Autodesk Inventor part; units mm, degrees
(part 2 of 5)
  line L413 (269.721, 22.163) -> (269.721, 35.9625) projected
  line L414 (269.721, 35.9625) -> (283.52, 35.9625) projected
  line L415 (269.721, 35.9625) -> (283.52, 35.9625) projected
  line L416 (279.888, 47.7132) -> (279.888, 41.4433) projected
  line L417 (279.888, 47.7132) -> (279.888, 41.4433) projected
  line L418 (280.713, 47.7132) -> (279.888, 47.7132) projected
  line L419 (280.713, 47.7132) -> (279.888, 47.7132) projected
  line L420 (302.57, 55.0125) -> (302.57, 41.2129) projected
  line L421 (302.57, 55.0125) -> (302.57, 41.2129) projected
  line L422 (280.713, 50.3135) -> (280.713, 47.7132) projected
  line L423 (280.713, 50.3135) -> (280.713, 47.7132) projected
  line L424 (279.888, 50.3135) -> (280.713, 50.3135) projected
  line L425 (279.888, 50.3135) -> (280.713, 50.3135) projected
  line L426 (279.888, 53.5421) -> (279.888, 50.3135) projected
  line L427 (279.888, 53.5421) -> (279.888, 50.3135) projected
  line L428 (288.771, 41.2129) -> (288.771, 55.0125) projected
  line L429 (288.771, 41.2129) -> (288.771, 55.0125) projected
  line L430 (288.771, 55.0125) -> (302.57, 55.0125) projected
  line L431 (288.771, 55.0125) -> (302.57, 55.0125) projected
  line L432 (302.57, 41.2129) -> (288.771, 41.2129) projected
  line L433 (302.57, 41.2129) -> (288.771, 41.2129) projected
  line L434 (305.398, 1.5696) -> (305.441, 1.7198) projected
  line L435 (305.278, 1.2788) -> (305.343, 1.4221) projected
  line L436 (305.114, 1.0115) -> (305.201, 1.1424) projected
  line L437 (305.343, 1.4221) -> (305.398, 1.5696) projected
  line L438 (305.016, 0.8875) -> (305.114, 1.0115) projected
  line L439 (305.441, 1.7198) -> (305.471, 1.8741) projected
  line L440 (305.471, 1.8741) -> (305.489, 2.0298) projected
  line L441 (305.489, 2.0298) -> (305.496, 2.1869) projected
  line L442 (305.016, 0.8875) -> (305.114, 1.0115) projected
  line L443 (305.016, 0.8875) -> (305.114, 1.0115) projected
  line L444 (305.016, 0.8875) -> (305.114, 1.0115) projected
  line L445 (305.114, 1.0115) -> (305.201, 1.1424) projected
  line L446 (305.114, 1.0115) -> (305.201, 1.1424) projected
  line L447 (305.114, 1.0115) -> (305.201, 1.1424) projected
  line L448 (305.201, 1.1424) -> (305.278, 1.2788) projected
  line L449 (305.201, 1.1424) -> (305.278, 1.2788) projected
  line L450 (305.201, 1.1424) -> (305.278, 1.2788) projected
  line L451 (305.278, 1.2788) -> (305.343, 1.4221) projected
  line L452 (305.278, 1.2788) -> (305.343, 1.4221) projected
  line L453 (305.278, 1.2788) -> (305.343, 1.4221) projected
  line L454 (305.343, 1.4221) -> (305.398, 1.5696) projected
  line L455 (305.343, 1.4221) -> (305.398, 1.5696) projected
  line L456 (305.343, 1.4221) -> (305.398, 1.5696) projected
  line L457 (305.398, 1.5696) -> (305.441, 1.7198) projected
  line L458 (305.398, 1.5696) -> (305.441, 1.7198) projected
  line L459 (305.398, 1.5696) -> (305.441, 1.7198) projected
  line L460 (305.441, 1.7198) -> (305.471, 1.8741) projected
  line L461 (305.441, 1.7198) -> (305.471, 1.8741) projected
  line L462 (305.441, 1.7198) -> (305.471, 1.8741) projected
  line L463 (305.471, 1.8741) -> (305.489, 2.0298) projected
  line L464 (305.471, 1.8741) -> (305.489, 2.0299) projected
  line L465 (305.471, 1.8741) -> (305.489, 2.0298) projected
  line L466 (305.489, 2.0298) -> (305.496, 2.1869) projected
  line L467 (305.489, 2.0299) -> (305.496, 2.1869) projected
  line L468 (305.489, 2.0298) -> (305.496, 2.187) projected
  line L469 (304.115, 0.2853) -> (304.261, 0.339) projected
  line L470 (250.671, 16.9127) -> (264.47, 16.9127) projected
  line L471 (250.671, 16.9127) -> (264.47, 16.9127) projected
  line L472 (264.47, 16.9127) -> (264.47, 3.113) projected
  line L473 (264.47, 16.9127) -> (264.47, 3.113) projected
  line L474 (264.47, 3.113) -> (250.671, 3.113) projected
  line L475 (264.47, 3.113) -> (250.671, 3.113) projected
  line L476 (269.721, 16.9127) -> (283.52, 16.9127) projected
  line L477 (269.721, 16.9127) -> (283.52, 16.9127) projected
  line L478 (283.52, 16.9127) -> (283.52, 3.113) projected
  line L479 (283.52, 3.113) -> (269.721, 3.113) projected
  line L480 (283.52, 3.113) -> (269.721, 3.113) projected
  line L481 (269.721, 3.113) -> (269.721, 16.9127) projected
  line L482 (269.721, 3.113) -> (269.721, 16.9127) projected
  line L483 (283.52, 16.9127) -> (283.52, 3.113) projected
  line L484 (243.527, 35.9625) -> (257.327, 35.9625) projected
  line L485 (243.527, 35.9625) -> (257.327, 35.9625) projected
  line L486 (257.327, 35.9625) -> (257.327, 22.163) projected
  line L487 (257.327, 35.9625) -> (257.327, 22.163) projected
  line L488 (257.327, 22.163) -> (243.527, 22.163) projected
  line L489 (233.514, 16.9127) -> (233.514, 3.113) projected
  line L490 (233.514, 16.9127) -> (233.514, 3.113) projected
  line L491 (257.327, 22.163) -> (243.527, 22.163) projected
  line L492 (250.671, 3.113) -> (250.671, 16.9127) projected
  line L493 (250.671, 3.113) -> (250.671, 16.9127) projected
  line L494 (233.514, 3.113) -> (219.713, 3.113) projected
  line L495 (233.514, 3.113) -> (219.713, 3.113) projected
  line L496 (219.713, 3.113) -> (219.713, 16.9127) projected
  line L497 (219.713, 3.113) -> (219.713, 16.9127) projected
  line L498 (243.527, 22.163) -> (243.527, 35.9625) projected
  line L499 (243.527, 22.163) -> (243.527, 35.9625) projected
  line L500 (219.713, 16.9127) -> (233.514, 16.9127) projected
  line L501 (219.713, 16.9127) -> (233.514, 16.9127) projected
  line L502 (231.133, 35.9625) -> (231.133, 22.163) projected
  line L503 (231.133, 35.9625) -> (231.133, 22.163) projected
  line L504 (231.133, 22.163) -> (217.333, 22.163) projected
  line L505 (231.133, 22.163) -> (217.333, 22.163) projected
  line L506 (217.333, 35.9625) -> (231.133, 35.9625) projected
  line L507 (217.333, 35.9625) -> (231.133, 35.9625) projected
  line L508 (217.333, 22.163) -> (217.333, 35.9625) projected
  line L509 (217.333, 22.163) -> (217.333, 35.9625) projected
  line L510 (241.146, 60.2629) -> (241.146, 74.0625) projected
  line L511 (1.6288, 119.796) -> (1.4759, 119.753) projected
  line L512 (1.4759, 119.753) -> (1.3298, 119.698) projected
  line L513 (1.3298, 119.698) -> (1.1879, 119.633) projected
  line L514 (1.3298, 119.698) -> (1.1879, 119.633) projected
  line L515 (1.1879, 119.633) -> (1.0501, 119.556) projected
  line L516 (1.1879, 119.633) -> (1.0501, 119.556) projected
  line L517 (1.0501, 119.556) -> (0.9192, 119.469) projected
  line L518 (1.0501, 119.556) -> (0.9192, 119.469) projected
  line L519 (1.4759, 119.753) -> (1.3298, 119.698) projected
  line L520 (1.6288, 119.796) -> (1.4759, 119.753) projected
  line L521 (0.9192, 119.469) -> (0.7965, 119.371) projected
  line L522 (0.7965, 119.371) -> (0.6808, 119.265) projected
  line L523 (0.7965, 119.371) -> (0.6808, 119.265) projected
  line L524 (0.6808, 119.265) -> (0.5746, 119.149) projected
  line L525 (0.6808, 119.265) -> (0.5746, 119.149) projected
  line L526 (0.5746, 119.149) -> (0.4768, 119.025) projected
  line L527 (0.5746, 119.149) -> (0.4768, 119.025) projected
  line L528 (0.4768, 119.025) -> (0.39, 118.894) projected
  line L529 (0.4768, 119.025) -> (0.39, 118.894) projected
  line L530 (303.496, 119.849) -> (2.096, 119.849) projected
  line L531 (303.496, 119.849) -> (2.096, 119.849) projected
  line L532 (2.096, 119.849) -> (1.9389, 119.844) projected
  line L533 (2.096, 119.849) -> (1.9389, 119.844) projected
  line L534 (1.9389, 119.844) -> (1.7818, 119.826) projected
  line L535 (1.9389, 119.844) -> (1.7818, 119.826) projected
  line L536 (1.7818, 119.826) -> (1.6288, 119.796) projected
  line L537 (1.7818, 119.826) -> (1.6288, 119.796) projected
  line L538 (303.496, 119.849) -> (2.096, 119.849) projected
  line L539 (303.496, 119.849) -> (2.096, 119.849) projected
  line L540 (303.496, 119.849) -> (2.096, 119.849) projected
  line L541 (2.096, 119.849) -> (1.9389, 119.844) projected
  line L542 (1.9389, 119.844) -> (1.7818, 119.826) projected
  line L543 (1.7818, 119.826) -> (1.6288, 119.796) projected
  line L544 (1.6288, 119.796) -> (1.4759, 119.753) projected
  line L545 (1.4759, 119.753) -> (1.3298, 119.698) projected
  line L546 (1.3298, 119.698) -> (1.1879, 119.633) projected
  line L547 (1.1879, 119.633) -> (1.0501, 119.556) projected
  line L548 (1.0501, 119.556) -> (0.9192, 119.469) projected
  line L549 (0.9192, 119.469) -> (0.7965, 119.371) projected
  line L550 (0.7965, 119.371) -> (0.6808, 119.265) projected
  line L551 (0.6808, 119.265) -> (0.5746, 119.149) projected
  line L552 (0.5746, 119.149) -> (0.4768, 119.025) projected
  line L553 (0.4768, 119.025) -> (0.39, 118.894) projected
  line L554 (0.39, 118.894) -> (0.3128, 118.758) projected
  line L555 (0.3128, 118.758) -> (0.248, 118.616) projected
  line L556 (0.248, 118.616) -> (0.1929, 118.468) projected
  line L557 (0.1929, 118.468) -> (0.1502, 118.317) projected
  line L558 (0.1502, 118.317) -> (0.1199, 118.163) projected
  line L559 (0.1199, 118.163) -> (0.102, 118.007) projected
  line L560 (0.102, 118.007) -> (0.0951, 117.85) projected
  line L561 (0.0951, 117.85) -> (0.0951, 2.187) projected
  line L562 (0.0951, 2.187) -> (0.102, 2.0298) projected
  line L563 (0.102, 2.0298) -> (0.1199, 1.8741) projected
  line L564 (0.1199, 1.8741) -> (0.1502, 1.7198) projected
  line L565 (0.1502, 1.7198) -> (0.1929, 1.5696) projected
  line L566 (0.1929, 1.5696) -> (0.248, 1.4221) projected
  line L567 (0.248, 1.4221) -> (0.3128, 1.2788) projected
  line L568 (0.3128, 1.2788) -> (0.39, 1.1424) projected
  line L569 (0.39, 1.1424) -> (0.4768, 1.0115) projected
  line L570 (0.4768, 1.0115) -> (0.5746, 0.8875) projected
  line L571 (0.5746, 0.8875) -> (0.6808, 0.7731) projected
  line L572 (0.6808, 0.7731) -> (0.7965, 0.6656) projected
  line L573 (0.7965, 0.6656) -> (0.9192, 0.5691) projected
  line L574 (0.9192, 0.5691) -> (1.0501, 0.4823) projected
  line L575 (1.0501, 0.4823) -> (1.1879, 0.4051) projected
  line L576 (1.1879, 0.4051) -> (1.3298, 0.339) projected
  line L577 (1.3298, 0.339) -> (1.4759, 0.2853) projected
  line L578 (1.4759, 0.2853) -> (1.6288, 0.2425) projected
  line L579 (1.6288, 0.2425) -> (1.7818, 0.2122) projected
  line L580 (1.7818, 0.2122) -> (1.9389, 0.1929) projected
  line L581 (1.9389, 0.1929) -> (2.096, 0.1874) projected
  line L582 (2.096, 0.1874) -> (303.496, 0.1874) projected
  line L583 (303.496, 0.1874) -> (303.652, 0.1929) projected
  line L584 (303.652, 0.1929) -> (303.808, 0.2122) projected
  line L585 (303.808, 0.2122) -> (303.962, 0.2425) projected
  line L586 (303.962, 0.2425) -> (304.115, 0.2853) projected
  line L587 (304.115, 0.2853) -> (304.261, 0.339) projected
  line L588 (304.261, 0.339) -> (304.403, 0.4051) projected
  line L589 (304.403, 0.4051) -> (304.541, 0.4823) projected
  line L590 (304.541, 0.4823) -> (304.672, 0.5691) projected
  line L591 (304.672, 0.5691) -> (304.794, 0.6656) projected
  line L592 (304.794, 0.6656) -> (304.91, 0.7731) projected
  line L593 (304.91, 0.7731) -> (305.016, 0.8875) projected
  line L594 (305.016, 0.8875) -> (305.114, 1.0115) projected
  line L595 (305.114, 1.0115) -> (305.201, 1.1424) projected
  line L596 (305.201, 1.1424) -> (305.278, 1.2788) projected
  line L597 (305.278, 1.2788) -> (305.343, 1.4221) projected
  line L598 (305.343, 1.4221) -> (305.398, 1.5696) projected
  line L599 (305.398, 1.5696) -> (305.441, 1.7198) projected
  line L600 (305.441, 1.7198) -> (305.471, 1.8741) projected
  line L601 (305.471, 1.8741) -> (305.489, 2.0298) projected
  line L602 (305.489, 2.0298) -> (305.496, 2.187) projected
  line L603 (305.496, 2.187) -> (305.496, 117.85) projected
  line L604 (305.496, 117.85) -> (305.489, 118.007) projected
  line L605 (305.489, 118.007) -> (305.471, 118.163) projected
  line L606 (305.471, 118.163) -> (305.441, 118.317) projected
  line L607 (305.441, 118.317) -> (305.398, 118.468) projected
  line L608 (305.398, 118.468) -> (305.343, 118.616) projected
  line L609 (305.343, 118.616) -> (305.278, 118.758) projected
  line L610 (305.278, 118.758) -> (305.201, 118.894) projected
  line L611 (305.201, 118.894) -> (305.114, 119.025) projected
  line L612 (305.114, 119.025) -> (305.016, 119.149) projected
  line L613 (305.016, 119.149) -> (304.91, 119.265) projected
  line L614 (304.91, 119.265) -> (304.794, 119.371) projected
  line L615 (304.794, 119.371) -> (304.672, 119.469) projected
  line L616 (304.672, 119.469) -> (304.541, 119.556) projected
  line L617 (304.541, 119.556) -> (304.403, 119.633) projected
  line L618 (304.403, 119.633) -> (304.261, 119.698) projected
  line L619 (304.261, 119.698) -> (304.115, 119.753) projected
  line L620 (304.115, 119.753) -> (303.962, 119.796) projected
  line L621 (303.962, 119.796) -> (303.808, 119.826) projected
  line L622 (303.808, 119.826) -> (303.652, 119.844) projected
  line L623 (303.652, 119.844) -> (303.496, 119.849) projected
  line L624 (288.771, 79.3129) -> (288.771, 93.1125) projected
  line L625 (288.771, 93.1125) -> (302.57, 93.1125) projected
  line L626 (302.57, 93.1125) -> (302.57, 79.3129) projected
  line L627 (302.57, 79.3129) -> (288.771, 79.3129) projected
  line L628 (243.527, 35.9625) -> (257.327, 35.9625) projected
  line L629 (257.327, 35.9625) -> (257.327, 22.163) projected
  line L630 (257.327, 22.163) -> (243.527, 22.163) projected
  line L631 (243.527, 22.163) -> (243.527, 35.9625) projected
  line L632 (302.57, 60.2629) -> (288.771, 60.2629) projected
  line L633 (288.771, 60.2629) -> (288.771, 74.0625) projected
  line L634 (288.771, 74.0625) -> (302.57, 74.0625) projected
  line L635 (302.57, 74.0625) -> (302.57, 60.2629) projected
  line L636 (250.671, 16.9127) -> (264.47, 16.9127) projected
  line L637 (264.47, 16.9127) -> (264.47, 3.113) projected
  line L638 (264.47, 3.113) -> (250.671, 3.113) projected
  line L639 (250.671, 3.113) -> (250.671, 16.9127) projected
  line L640 (219.713, 16.9127) -> (233.514, 16.9127) projected
  line L641 (233.514, 16.9127) -> (233.514, 3.113) projected
  line L642 (233.514, 3.113) -> (219.713, 3.113) projected
  line L643 (219.713, 3.113) -> (219.713, 16.9127) projected
  line L644 (302.57, 41.2129) -> (288.771, 41.2129) projected
  line L645 (288.771, 41.2129) -> (288.771, 55.0125) projected
  line L646 (288.771, 55.0125) -> (302.57, 55.0125) projected
  line L647 (302.57, 55.0125) -> (302.57, 41.2129) projected
  line L648 (288.771, 16.9127) -> (302.57, 16.9127) projected
  line L649 (302.57, 16.9127) -> (302.57, 3.113) projected
  line L650 (302.57, 3.113) -> (288.771, 3.113) projected
  line L651 (288.771, 3.113) -> (288.771, 16.9127) projected
  line L652 (269.721, 16.9127) -> (283.52, 16.9127) projected
  line L653 (283.52, 16.9127) -> (283.52, 3.113) projected
  line L654 (283.52, 3.113) -> (269.721, 3.113) projected
  line L655 (269.721, 3.113) -> (269.721, 16.9127) projected
  line L656 (283.52, 22.163) -> (269.721, 22.163) projected
  line L657 (269.721, 22.163) -> (269.721, 35.9625) projected
  line L658 (269.721, 35.9625) -> (283.52, 35.9625) projected
  line L659 (283.52, 35.9625) -> (283.52, 22.163) projected
  line L660 (288.771, 35.9625) -> (302.57, 35.9625) projected
  line L661 (302.57, 35.9625) -> (302.57, 22.163) projected
  line L662 (302.57, 22.163) -> (288.771, 22.163) projected
  line L663 (288.771, 22.163) -> (288.771, 35.9625) projected
  line L664 (59.6829, 35.9625) -> (59.6829, 22.163) projected
  line L665 (59.6829, 22.163) -> (45.8833, 22.163) projected
  line L666 (45.8833, 22.163) -> (45.8833, 35.9625) projected
  line L667 (45.8833, 35.9625) -> (59.6829, 35.9625) projected
  line L668 (5.4019, 16.9127) -> (19.2016, 16.9127) projected
  line L669 (19.2016, 16.9127) -> (19.2016, 3.113) projected
  line L670 (19.2016, 3.113) -> (5.4019, 3.113) projected
  line L671 (5.4019, 3.113) -> (5.4019, 16.9127) projected
  line L672 (29.213, 16.9127) -> (43.0142, 16.9127) projected
  line L673 (43.0142, 16.9127) -> (43.0142, 3.113) projected
  line L674 (43.0142, 3.113) -> (29.213, 3.113) projected
  line L675 (29.213, 3.113) -> (29.213, 16.9127) projected
  line L676 (145.408, 55.0125) -> (145.408, 41.2129) projected
  line L677 (145.408, 41.2129) -> (131.608, 41.2129) projected
  line L678 (131.608, 41.2129) -> (131.608, 55.0125) projected
  line L679 (131.608, 55.0125) -> (145.408, 55.0125) projected
  line L680 (164.458, 41.2129) -> (150.658, 41.2129) projected
  line L681 (150.658, 41.2129) -> (150.658, 55.0125) projected
  line L682 (150.658, 55.0125) -> (164.458, 55.0125) projected
  line L683 (164.458, 55.0125) -> (164.458, 41.2129) projected
  line L684 (273.995, 103.125) -> (260.196, 103.125) projected
  line L685 (260.196, 103.125) -> (260.196, 116.926) projected
  line L686 (260.196, 116.926) -> (273.995, 116.926) projected
  line L687 (273.995, 116.926) -> (273.995, 103.125) projected
  line L688 (241.146, 74.0625) -> (254.945, 74.0625) projected
  line L689 (254.945, 74.0625) -> (254.945, 60.2629) projected
  line L690 (254.945, 60.2629) -> (241.146, 60.2629) projected
  line L691 (241.146, 60.2629) -> (241.146, 74.0625) projected
  line L692 (254.945, 103.125) -> (241.146, 103.125) projected
  line L693 (241.146, 103.125) -> (241.146, 116.926) projected
  line L694 (241.146, 116.926) -> (254.945, 116.926) projected
  line L695 (254.945, 116.926) -> (254.945, 103.125) projected
  line L696 (235.895, 103.125) -> (222.096, 103.125) projected
  line L697 (222.096, 103.125) -> (222.096, 116.926) projected
  line L698 (222.096, 116.926) -> (235.895, 116.926) projected
  line L699 (235.895, 116.926) -> (235.895, 103.125) projected
  line L700 (245.42, 79.3129) -> (231.621, 79.3129) projected
  line L701 (231.621, 79.3129) -> (231.621, 93.1125) projected
  line L702 (231.621, 93.1125) -> (245.42, 93.1125) projected
  line L703 (245.42, 93.1125) -> (245.42, 79.3129) projected
  line L704 (226.37, 79.3129) -> (212.571, 79.3129) projected
  line L705 (212.571, 79.3129) -> (212.571, 93.1125) projected
  line L706 (212.571, 93.1125) -> (226.37, 93.1125) projected
  line L707 (226.37, 93.1125) -> (226.37, 79.3129) projected
  line L708 (217.333, 35.9625) -> (231.133, 35.9625) projected
  line L709 (231.133, 35.9625) -> (231.133, 22.163) projected
  line L710 (231.133, 22.163) -> (217.333, 22.163) projected
  line L711 (217.333, 22.163) -> (217.333, 35.9625) projected
  line L712 (198.283, 35.9625) -> (212.083, 35.9625) projected
  line L713 (212.083, 35.9625) -> (212.083, 22.163) projected
  line L714 (212.083, 22.163) -> (198.283, 22.163) projected
  line L715 (198.283, 22.163) -> (198.283, 35.9625) projected
  line L716 (235.895, 60.2629) -> (222.096, 60.2629) projected
  line L717 (222.096, 60.2629) -> (222.096, 74.0625) projected
  line L718 (222.096, 74.0625) -> (235.895, 74.0625) projected
  line L719 (235.895, 74.0625) -> (235.895, 60.2629) projected
  line L720 (193.033, 103.125) -> (179.233, 103.125) projected
  line L721 (179.233, 103.125) -> (179.233, 116.926) projected
  line L722 (179.233, 116.926) -> (193.033, 116.926) projected
  line L723 (193.033, 116.926) -> (193.033, 103.125) projected
  line L724 (216.845, 103.125) -> (203.046, 103.125) projected
  line L725 (203.046, 103.125) -> (203.046, 116.926) projected
  line L726 (203.046, 116.926) -> (216.845, 116.926) projected
  line L727 (216.845, 116.926) -> (216.845, 103.125) projected
  line L728 (216.845, 74.0625) -> (216.845, 60.2629) projected
  line L729 (216.845, 60.2629) -> (203.046, 60.2629) projected
  line L730 (203.046, 60.2629) -> (203.046, 74.0625) projected
  line L731 (203.046, 74.0625) -> (216.845, 74.0625) projected
  line L732 (207.32, 79.3129) -> (193.521, 79.3129) projected
  line L733 (193.521, 79.3129) -> (193.521, 93.1125) projected
  line L734 (193.521, 93.1125) -> (207.32, 93.1125) projected
  line L735 (207.32, 93.1125) -> (207.32, 79.3129) projected
  line L736 (188.27, 79.3129) -> (174.471, 79.3129) projected
  line L737 (174.471, 79.3129) -> (174.471, 93.1125) projected
  line L738 (174.471, 93.1125) -> (188.27, 93.1125) projected
  line L739 (188.27, 93.1125) -> (188.27, 79.3129) projected
  line L740 (183.508, 55.0125) -> (183.508, 41.2129) projected
  line L741 (183.508, 41.2129) -> (169.708, 41.2129) projected
  line L742 (169.708, 41.2129) -> (169.708, 55.0125) projected
  line L743 (169.708, 55.0125) -> (183.508, 55.0125) projected
  line L744 (197.795, 60.2629) -> (183.996, 60.2629) projected
  line L745 (183.996, 60.2629) -> (183.996, 74.0625) projected
  line L746 (183.996, 74.0625) -> (197.795, 74.0625) projected
  line L747 (197.795, 74.0625) -> (197.795, 60.2629) projected
  line L748 (178.745, 74.0625) -> (178.745, 60.2629) projected
  line L749 (178.745, 60.2629) -> (164.946, 60.2629) projected
  line L750 (164.946, 60.2629) -> (164.946, 74.0625) projected
  line L751 (164.946, 74.0625) -> (178.745, 74.0625) projected
  line L752 (154.933, 103.125) -> (141.133, 103.125) projected
  line L753 (141.133, 103.125) -> (141.133, 116.926) projected
  line L754 (141.133, 116.926) -> (154.933, 116.926) projected
  line L755 (154.933, 116.926) -> (154.933, 103.125) projected
  line L756 (173.983, 103.125) -> (160.183, 103.125) projected
  line L757 (160.183, 103.125) -> (160.183, 116.926) projected
  line L758 (160.183, 116.926) -> (173.983, 116.926) projected
  line L759 (173.983, 116.926) -> (173.983, 103.125) projected
  line L760 (169.22, 79.3129) -> (155.421, 79.3129) projected
  line L761 (155.421, 79.3129) -> (155.421, 93.1125) projected
  line L762 (155.421, 93.1125) -> (169.22, 93.1125) projected
  line L763 (169.22, 93.1125) -> (169.22, 79.3129) projected
  line L764 (150.17, 79.3129) -> (136.371, 79.3129) projected
  line L765 (136.371, 79.3129) -> (136.371, 93.1125) projected
  line L766 (136.371, 93.1125) -> (150.17, 93.1125) projected
  line L767 (150.17, 93.1125) -> (150.17, 79.3129) projected
  line L768 (260.196, 79.3129) -> (260.196, 84.0133) projected
  line L769 (260.196, 84.0133) -> (258.47, 84.0133) projected
  line L770 (258.47, 84.0133) -> (258.47, 79.5433) projected
  line L771 (258.47, 79.5433) -> (256.745, 79.5433) projected
  line L772 (256.745, 79.5433) -> (256.745, 78.3428) projected
  line L773 (256.745, 78.3428) -> (253.646, 78.3428) projected
  line L774 (253.646, 78.3428) -> (253.646, 79.5433) projected
  line L775 (253.646, 79.5433) -> (251.92, 79.5433) projected
  line L776 (251.92, 79.5433) -> (251.92, 85.8132) projected
  line L777 (251.92, 85.8132) -> (251.095, 85.8132) projected
  line L778 (251.095, 85.8132) -> (251.095, 88.4135) projected
  line L779 (251.095, 88.4135) -> (251.92, 88.4135) projected
  line L780 (251.92, 88.4135) -> (251.92, 91.6421) projected
  line L781 (251.92, 91.6421) -> (258.47, 91.6421) projected
  line L782 (258.47, 91.6421) -> (258.47, 88.4135) projected
  line L783 (258.47, 88.4135) -> (260.196, 88.4135) projected
  line L784 (260.196, 88.4135) -> (260.196, 93.1125) projected
  line L785 (260.196, 93.1125) -> (273.995, 93.1125) projected
  line L786 (273.995, 93.1125) -> (273.995, 88.4135) projected
  line L787 (273.995, 88.4135) -> (275.721, 88.4135) projected
  line L788 (275.721, 88.4135) -> (275.721, 91.6421) projected
  line L789 (275.721, 91.6421) -> (282.271, 91.6421) projected
  line L790 (282.271, 91.6421) -> (282.271, 88.4135) projected
  line L791 (282.271, 88.4135) -> (283.096, 88.4135) projected
  line L792 (283.096, 88.4135) -> (283.096, 85.8132) projected
  line L793 (283.096, 85.8132) -> (282.271, 85.8132) projected
  line L794 (282.271, 85.8132) -> (282.271, 79.5433) projected
  line L795 (282.271, 79.5433) -> (280.545, 79.5433) projected
  line L796 (280.545, 79.5433) -> (280.545, 78.3428) projected
  line L797 (280.545, 78.3428) -> (277.446, 78.3428) projected
  line L798 (277.446, 78.3428) -> (277.446, 79.5433) projected
  line L799 (277.446, 79.5433) -> (275.721, 79.5433) projected
  line L800 (275.721, 79.5433) -> (275.721, 84.0133) projected
  line L801 (275.721, 84.0133) -> (273.995, 84.0133) projected
  line L802 (273.995, 84.0133) -> (273.995, 79.3129) projected
  line L803 (273.995, 79.3129) -> (260.196, 79.3129) projected
  line L804 (278.758, 60.2629) -> (264.958, 60.2629) projected
  line L805 (264.958, 60.2629) -> (264.958, 74.0625) projected
  line L806 (264.958, 74.0625) -> (278.758, 74.0625) projected
  line L807 (278.758, 74.0625) -> (278.758, 60.2629) projected
  line L808 (257.813, 55.0125) -> (271.614, 55.0125) projected
  line L809 (271.614, 55.0125) -> (271.614, 50.3135) projected
  line L810 (271.614, 50.3135) -> (273.338, 50.3135) projected
  line L811 (273.338, 50.3135) -> (273.338, 53.5421) projected
  line L812 (273.338, 53.5421) -> (279.888, 53.5421) projected
  line L813 (279.888, 53.5421) -> (279.888, 50.3135) projected
  line L814 (279.888, 50.3135) -> (280.713, 50.3135) projected
  line L815 (280.713, 50.3135) -> (280.713, 47.7132) projected
  line L816 (280.713, 47.7132) -> (279.888, 47.7132) projected
  line L817 (279.888, 47.7132) -> (279.888, 41.4433) projected
  line L818 (279.888, 41.4433) -> (278.164, 41.4433) projected
  line L819 (278.164, 41.4433) -> (278.164, 40.2428) projected
  line L820 (278.164, 40.2428) -> (275.063, 40.2428) projected
  line L821 (275.063, 40.2428) -> (275.063, 41.4433) projected
  line L822 (275.063, 41.4433) -> (273.338, 41.4433) projected
  line L823 (273.338, 41.4433) -> (273.338, 45.9133) projected
  line L824 (273.338, 45.9133) -> (271.614, 45.9133) projected
  line L825 (271.614, 45.9133) -> (271.614, 41.2129) projected
  line L826 (271.614, 41.2129) -> (257.813, 41.2129) projected
  line L827 (257.813, 41.2129) -> (257.813, 45.9133) projected
  line L828 (257.813, 45.9133) -> (256.089, 45.9133) projected
  line L829 (256.089, 45.9133) -> (256.089, 41.4433) projected
  line L830 (256.089, 41.4433) -> (254.362, 41.4433) projected
  line L831 (254.362, 41.4433) -> (254.362, 40.2428) projected
  line L832 (254.362, 40.2428) -> (251.263, 40.2428) projected
  line L833 (251.263, 40.2428) -> (251.263, 41.4433) projected
  line L834 (251.263, 41.4433) -> (249.538, 41.4433) projected
  line L835 (249.538, 41.4433) -> (249.538, 47.7132) projected
  line L836 (249.538, 47.7132) -> (248.714, 47.7132) projected
  line L837 (248.714, 47.7132) -> (248.714, 50.3135) projected
  line L838 (248.714, 50.3135) -> (249.538, 50.3135) projected
  line L839 (249.538, 50.3135) -> (249.538, 53.5421) projected
  line L840 (249.538, 53.5421) -> (256.089, 53.5421) projected
  line L841 (256.089, 53.5421) -> (256.089, 50.3135) projected
  line L842 (256.089, 50.3135) -> (257.813, 50.3135) projected
  line L843 (257.813, 50.3135) -> (257.813, 55.0125) projected
  line L844 (226.858, 41.2129) -> (226.858, 55.0125) projected
  line L845 (226.858, 55.0125) -> (240.658, 55.0125) projected
  line L846 (240.658, 55.0125) -> (240.658, 41.2129) projected
  line L847 (240.658, 41.2129) -> (226.858, 41.2129) projected
  line L848 (221.608, 55.0125) -> (221.608, 41.2129) projected
  line L849 (221.608, 41.2129) -> (207.808, 41.2129) projected
  line L850 (207.808, 41.2129) -> (207.808, 55.0125) projected
  line L851 (207.808, 55.0125) -> (221.608, 55.0125) projected
  line L852 (202.558, 41.2129) -> (188.758, 41.2129) projected
  line L853 (188.758, 41.2129) -> (188.758, 55.0125) projected
  line L854 (188.758, 55.0125) -> (202.558, 55.0125) projected
  line L855 (202.558, 55.0125) -> (202.558, 41.2129) projected
  line L856 (122.083, 35.9625) -> (135.883, 35.9625) projected
  line L857 (135.883, 35.9625) -> (135.883, 22.163) projected
  line L858 (135.883, 22.163) -> (122.083, 22.163) projected
  line L859 (122.083, 22.163) -> (122.083, 35.9625) projected
  line L860 (195.902, 16.9127) -> (209.702, 16.9127) projected
  line L861 (209.702, 16.9127) -> (209.702, 3.113) projected
  line L862 (209.702, 3.113) -> (195.902, 3.113) projected
  line L863 (195.902, 3.113) -> (195.902, 16.9127) projected
  line L864 (193.033, 22.163) -> (179.233, 22.163) projected
  line L865 (179.233, 22.163) -> (179.233, 35.9625) projected
  line L866 (179.233, 35.9625) -> (193.033, 35.9625) projected
  line L867 (193.033, 35.9625) -> (193.033, 22.163) projected
  line L868 (160.183, 22.163) -> (160.183, 35.9625) projected
  line L869 (160.183, 35.9625) -> (173.983, 35.9625) projected
  line L870 (173.983, 35.9625) -> (173.983, 22.163) projected
  line L871 (173.983, 22.163) -> (160.183, 22.163) projected
  line L872 (141.133, 22.163) -> (141.133, 35.9625) projected
  line L873 (141.133, 35.9625) -> (154.933, 35.9625) projected
  line L874 (154.933, 35.9625) -> (154.933, 22.163) projected
  line L875 (154.933, 22.163) -> (141.133, 22.163) projected
  line L876 (73.9704, 103.125) -> (60.1694, 103.125) projected
  line L877 (60.1694, 103.125) -> (60.1694, 116.926) projected
  line L878 (60.1694, 116.926) -> (73.9704, 116.926) projected
  line L879 (73.9704, 116.926) -> (73.9704, 103.125) projected
  line L880 (131.12, 79.3129) -> (117.321, 79.3129) projected
  line L881 (117.321, 79.3129) -> (117.321, 93.1125) projected
  line L882 (117.321, 93.1125) -> (131.12, 93.1125) projected
  line L883 (131.12, 93.1125) -> (131.12, 79.3129) projected
  line L884 (112.07, 79.3129) -> (98.2694, 79.3129) projected
  line L885 (98.2694, 79.3129) -> (98.2694, 93.1125) projected
  line L886 (98.2694, 93.1125) -> (112.07, 93.1125) projected
  line L887 (112.07, 93.1125) -> (112.07, 79.3129) projected
  line L888 (140.645, 74.0625) -> (140.645, 60.2629) projected
  line L889 (140.645, 60.2629) -> (126.846, 60.2629) projected
  line L890 (126.846, 60.2629) -> (126.846, 74.0625) projected
  line L891 (126.846, 74.0625) -> (140.645, 74.0625) projected
  line L892 (145.896, 74.0625) -> (159.695, 74.0625) projected
  line L893 (159.695, 74.0625) -> (159.695, 60.2629) projected
  line L894 (159.695, 60.2629) -> (145.896, 60.2629) projected
  line L895 (145.896, 60.2629) -> (145.896, 74.0625) projected
  line L896 (93.0204, 103.125) -> (79.2194, 103.125) projected
  line L897 (79.2194, 103.125) -> (79.2194, 116.926) projected
  line L898 (79.2194, 116.926) -> (93.0204, 116.926) projected
  line L899 (93.0204, 116.926) -> (93.0204, 103.125) projected
  line L900 (112.558, 41.2129) -> (112.558, 55.0125) projected
  line L901 (112.558, 55.0125) -> (126.358, 55.0125) projected
  line L902 (126.358, 55.0125) -> (126.358, 41.2129) projected
  line L903 (126.358, 41.2129) -> (112.558, 41.2129) projected
  line L904 (54.919, 103.125) -> (41.1208, 103.125) projected
  line L905 (41.1208, 103.125) -> (41.1208, 116.926) projected
  line L906 (41.1208, 116.926) -> (54.919, 116.926) projected
  line L907 (54.919, 116.926) -> (54.919, 103.125) projected
  line L908 (102.545, 74.0625) -> (102.545, 60.2629) projected
  line L909 (102.545, 60.2629) -> (88.7444, 60.2629) projected
  line L910 (88.7444, 60.2629) -> (88.7444, 74.0625) projected
  line L911 (88.7444, 74.0625) -> (102.545, 74.0625) projected
  line L912 (107.794, 60.2629) -> (107.794, 74.0625) projected
  line L913 (107.794, 74.0625) -> (121.595, 74.0625) projected
  line L914 (121.595, 74.0625) -> (121.595, 60.2629) projected
  line L915 (121.595, 60.2629) -> (107.794, 60.2629) projected
  line L916 (79.2194, 79.3129) -> (79.2194, 93.1125) projected
  line L917 (79.2194, 93.1125) -> (93.0204, 93.1125) projected
  line L918 (93.0204, 93.1125) -> (93.0204, 79.3129) projected
  line L919 (93.0204, 79.3129) -> (79.2194, 79.3129) projected
  line L920 (73.9704, 79.3129) -> (60.1694, 79.3129) projected
  line L921 (60.1694, 79.3129) -> (60.1694, 93.1125) projected
  line L922 (60.1694, 93.1125) -> (73.9704, 93.1125) projected
  line L923 (73.9704, 93.1125) -> (73.9704, 79.3129) projected
  line L924 (50.6458, 74.0625) -> (64.4454, 74.0625) projected
  line L925 (64.4454, 74.0625) -> (64.4454, 60.2629) projected
  line L926 (64.4454, 60.2629) -> (50.6458, 60.2629) projected
  line L927 (50.6458, 60.2629) -> (50.6458, 74.0625) projected
  line L928 (83.4954, 60.2629) -> (69.6958, 60.2629) projected
  line L929 (69.6958, 60.2629) -> (69.6958, 74.0625) projected
  line L930 (69.6958, 74.0625) -> (83.4954, 74.0625) projected
  line L931 (83.4954, 74.0625) -> (83.4954, 60.2629) projected
  line L932 (74.4583, 41.2129) -> (74.4583, 55.0125) projected
  line L933 (74.4583, 55.0125) -> (88.2579, 55.0125) projected
  line L934 (88.2579, 55.0125) -> (88.2579, 41.2129) projected
  line L935 (88.2579, 41.2129) -> (74.4583, 41.2129) projected
  line L936 (41.1208, 79.3129) -> (41.1208, 93.1125) projected
  line L937 (41.1208, 93.1125) -> (54.919, 93.1125) projected
  line L938 (54.919, 93.1125) -> (54.919, 79.3129) projected
  line L939 (54.919, 79.3129) -> (41.1208, 79.3129) projected
  line L940 (107.308, 41.2129) -> (93.5083, 41.2129) projected
  line L941 (93.5083, 41.2129) -> (93.5083, 55.0125) projected
  line L942 (93.5083, 55.0125) -> (107.308, 55.0125) projected
  line L943 (107.308, 55.0125) -> (107.308, 41.2129) projected
  line L944 (103.033, 22.163) -> (103.033, 35.9625) projected
  line L945 (103.033, 35.9625) -> (116.833, 35.9625) projected
  line L946 (116.833, 35.9625) -> (116.833, 22.163) projected
  line L947 (116.833, 22.163) -> (103.033, 22.163) projected
  line L948 (97.7829, 35.9625) -> (97.7829, 22.163) projected
  line L949 (97.7829, 22.163) -> (83.9833, 22.163) projected
  line L950 (83.9833, 22.163) -> (83.9833, 35.9625) projected
  line L951 (83.9833, 35.9625) -> (97.7829, 35.9625) projected
  line L952 (16.8203, 103.125) -> (3.0193, 103.125) projected
  line L953 (3.0193, 103.125) -> (3.0193, 116.926) projected
  line L954 (3.0193, 116.926) -> (16.8203, 116.926) projected
  line L955 (16.8203, 116.926) -> (16.8203, 103.125) projected
  line L956 (16.8203, 79.3129) -> (3.0193, 79.3129) projected
  line L957 (3.0193, 79.3129) -> (3.0193, 93.1125) projected
  line L958 (3.0193, 93.1125) -> (16.8203, 93.1125) projected
  line L959 (16.8203, 93.1125) -> (16.8203, 79.3129) projected
  line L960 (35.8704, 79.3129) -> (22.0707, 79.3129) projected
  line L961 (22.0707, 79.3129) -> (22.0707, 93.1125) projected
  line L962 (22.0707, 93.1125) -> (35.8704, 93.1125) projected
  line L963 (35.8704, 93.1125) -> (35.8704, 79.3129) projected
  line L964 (31.5957, 60.2629) -> (31.5957, 74.0625) projected
  line L965 (31.5957, 74.0625) -> (45.3954, 74.0625) projected
  line L966 (45.3954, 74.0625) -> (45.3954, 60.2629) projected
  line L967 (45.3954, 60.2629) -> (31.5957, 60.2629) projected
  line L968 (21.5828, 60.2629) -> (7.7832, 60.2629) projected
  line L969 (7.7832, 60.2629) -> (7.7832, 74.0625) projected
  line L970 (7.7832, 74.0625) -> (21.5828, 74.0625) projected
  line L971 (21.5828, 74.0625) -> (21.5828, 60.2629) projected
  line L972 (50.1579, 55.0125) -> (50.1579, 41.2129) projected
  line L973 (50.1579, 41.2129) -> (36.3583, 41.2129) projected
  line L974 (36.3583, 41.2129) -> (36.3583, 55.0125) projected
  line L975 (36.3583, 55.0125) -> (50.1579, 55.0125) projected
  line L976 (69.2079, 41.2129) -> (55.4083, 41.2129) projected
  line L977 (55.4083, 41.2129) -> (55.4083, 55.0125) projected
  line L978 (55.4083, 55.0125) -> (69.2079, 55.0125) projected
  line L979 (69.2079, 55.0125) -> (69.2079, 41.2129) projected
  line L980 (78.7329, 22.163) -> (64.9333, 22.163) projected
  line L981 (64.9333, 22.163) -> (64.9333, 35.9625) projected
  line L982 (64.9333, 35.9625) -> (78.7329, 35.9625) projected
  line L983 (78.7329, 35.9625) -> (78.7329, 22.163) projected
  line L984 (53.0271, 16.9127) -> (66.8267, 16.9127) projected
  line L985 (66.8267, 16.9127) -> (66.8267, 3.113) projected
  line L986 (66.8267, 3.113) -> (53.0271, 3.113) projected
  line L987 (53.0271, 3.113) -> (53.0271, 16.9127) projected
  line L988 (78.0881, 15.4423) -> (84.6391, 15.4423) projected
  line L989 (84.6391, 15.4423) -> (84.6391, 12.2136) projected
  line L990 (84.6391, 12.2136) -> (124.463, 12.2136) projected
  line L991 (124.463, 12.2136) -> (124.463, 16.9127) projected
  line L992 (124.463, 16.9127) -> (138.264, 16.9127) projected
  line L993 (138.264, 16.9127) -> (138.264, 12.2136) projected
  line L994 (138.264, 12.2136) -> (178.088, 12.2136) projected
  line L995 (178.088, 12.2136) -> (178.088, 15.4423) projected
  line L996 (178.088, 15.4423) -> (184.638, 15.4423) projected
  line L997 (184.638, 15.4423) -> (184.638, 12.2136) projected
  line L998 (184.638, 12.2136) -> (185.463, 12.2136) projected
  line L999 (185.463, 12.2136) -> (185.463, 9.6132) projected
  line L1000 (185.463, 9.6132) -> (184.638, 9.6132) projected
  line L1001 (184.638, 9.6132) -> (184.638, 3.3431) projected
  line L1002 (184.638, 3.3431) -> (182.914, 3.3431) projected
  line L1003 (182.914, 3.3431) -> (182.914, 2.1429) projected
  line L1004 (182.914, 2.1429) -> (179.813, 2.1429) projected
  line L1005 (179.813, 2.1429) -> (179.813, 3.3431) projected
  line L1006 (179.813, 3.3431) -> (178.088, 3.3431) projected
  line L1007 (178.088, 3.3431) -> (178.088, 7.8135) projected
  line L1008 (178.088, 7.8135) -> (138.264, 7.8135) projected
  line L1009 (138.264, 7.8135) -> (138.264, 3.113) projected
  line L1010 (138.264, 3.113) -> (124.463, 3.113) projected
  line L1011 (124.463, 3.113) -> (124.463, 7.8135) projected
  line L1012 (124.463, 7.8135) -> (84.6391, 7.8135) projected
  line L1013 (84.6391, 7.8135) -> (84.6391, 3.3431) projected
  line L1014 (84.6391, 3.3431) -> (82.9137, 3.3431) projected
  line L1015 (82.9137, 3.3431) -> (82.9137, 2.1429) projected
  line L1016 (82.9137, 2.1429) -> (79.8132, 2.1429) projected
  line L1017 (79.8132, 2.1429) -> (79.8132, 3.3431) projected
  line L1018 (79.8132, 3.3431) -> (78.0881, 3.3431) projected
  line L1019 (78.0881, 3.3431) -> (78.0881, 9.6132) projected
  line L1020 (78.0881, 9.6132) -> (77.264, 9.6132) projected
  line L1021 (77.264, 9.6132) -> (77.264, 12.2136) projected
  line L1022 (77.264, 12.2136) -> (78.0881, 12.2136) projected
  line L1023 (78.0881, 12.2136) -> (78.0881, 15.4423) projected
  line L1024 (23.9641, 55.0125) -> (23.9641, 41.2129) projected
  line L1025 (23.9641, 41.2129) -> (10.163, 41.2129) projected
  line L1026 (10.163, 41.2129) -> (10.163, 55.0125) projected
  line L1027 (10.163, 55.0125) -> (23.9641, 55.0125) projected
  line L1028 (28.7266, 35.9625) -> (28.7266, 31.2636) projected
  line L1029 (28.7266, 31.2636) -> (30.4519, 31.2636) projected
  line L1030 (30.4519, 31.2636) -> (30.4519, 34.4923) projected
  line L1031 (30.4519, 34.4923) -> (37.0018, 34.4923) projected
  line L1032 (37.0018, 34.4923) -> (37.0018, 31.2636) projected
  line L1033 (37.0018, 31.2636) -> (37.8273, 31.2636) projected
  line L1034 (37.8273, 31.2636) -> (37.8273, 28.6632) projected
  line L1035 (37.8273, 28.6632) -> (37.0018, 28.6632) projected
  line L1036 (37.0018, 28.6632) -> (37.0018, 22.3931) projected
  line L1037 (37.0018, 22.3931) -> (35.2764, 22.3931) projected
  line L1038 (35.2764, 22.3931) -> (35.2764, 21.1928) projected
  line L1039 (35.2764, 21.1928) -> (32.1758, 21.1928) projected
  line L1040 (32.1758, 21.1928) -> (32.1758, 22.3931) projected
  line L1041 (32.1758, 22.3931) -> (30.4519, 22.3931) projected
  line L1042 (30.4519, 22.3931) -> (30.4519, 26.8635) projected
  line L1043 (30.4519, 26.8635) -> (28.7266, 26.8635) projected
  line L1044 (28.7266, 26.8635) -> (28.7266, 22.163) projected
  line L1045 (28.7266, 22.163) -> (14.9269, 22.163) projected
  line L1046 (14.9269, 22.163) -> (14.9269, 26.8635) projected
  line L1047 (14.9269, 26.8635) -> (13.2016, 26.8635) projected
  line L1048 (13.2016, 26.8635) -> (13.2016, 22.3931) projected
  line L1049 (13.2016, 22.3931) -> (11.4763, 22.3931) projected
  line L1050 (11.4763, 22.3931) -> (11.4763, 21.1928) projected
  line L1051 (11.4763, 21.1928) -> (8.3771, 21.1928) projected
  line L1052 (8.3771, 21.1928) -> (8.3771, 22.3931) projected
  line L1053 (8.3771, 22.3931) -> (6.6518, 22.3931) projected
  line L1054 (6.6518, 22.3931) -> (6.6518, 28.6632) projected
  line L1055 (6.6518, 28.6632) -> (5.8263, 28.6632) projected
  line L1056 (5.8263, 28.6632) -> (5.8263, 31.2636) projected
  line L1057 (5.8263, 31.2636) -> (6.6518, 31.2636) projected
  line L1058 (6.6518, 31.2636) -> (6.6518, 34.4923) projected
  line L1059 (6.6518, 34.4923) -> (13.2016, 34.4923) projected
  line L1060 (13.2016, 34.4923) -> (13.2016, 31.2636) projected
  line L1061 (13.2016, 31.2636) -> (14.9269, 31.2636) projected
  line L1062 (14.9269, 31.2636) -> (14.9269, 35.9625) projected
  line L1063 (14.9269, 35.9625) -> (28.7266, 35.9625) projected
  line L1064 (98.2694, 116.926) -> (112.07, 116.926) projected
  line L1065 (112.07, 116.926) -> (112.07, 103.125) projected
  line L1066 (112.07, 103.125) -> (98.2694, 103.125) projected
  line L1067 (98.2694, 103.125) -> (98.2694, 116.926) projected
  line L1068 (135.883, 116.926) -> (135.883, 103.125) projected
  line L1069 (135.883, 103.125) -> (122.083, 103.125) projected
  line L1070 (122.083, 103.125) -> (122.083, 116.926) projected
  line L1071 (122.083, 116.926) -> (135.883, 116.926) projected
  line L1072 (303.496, 119.849) -> (2.096, 119.849) projected
  line L1073 (303.652, 119.844) -> (303.496, 119.849) projected
  line L1074 (303.808, 119.826) -> (303.652, 119.844) projected
  line L1075 (303.962, 119.796) -> (303.808, 119.826) projected
  line L1076 (304.115, 119.753) -> (303.962, 119.796) projected
  line L1077 (304.261, 119.698) -> (304.115, 119.753) projected
  line L1078 (304.403, 119.633) -> (304.261, 119.698) projected
  line L1079 (304.541, 119.556) -> (304.403, 119.633) projected
  line L1080 (304.672, 119.469) -> (304.541, 119.556) projected
  line L1081 (304.794, 119.371) -> (304.672, 119.469) projected
  line L1082 (304.91, 119.265) -> (304.794, 119.371) projected
  line L1083 (305.016, 119.149) -> (304.91, 119.265) projected
  line L1084 (305.114, 119.025) -> (305.016, 119.149) projected
  line L1085 (305.201, 118.894) -> (305.114, 119.025) projected
  line L1086 (305.278, 118.758) -> (305.201, 118.894) projected
  line L1087 (305.343, 118.616) -> (305.278, 118.758) projected
  line L1088 (305.398, 118.468) -> (305.343, 118.616) projected
  line L1089 (305.441, 118.317) -> (305.398, 118.468) projected
  line L1090 (305.471, 118.163) -> (305.441, 118.317) projected
  line L1091 (305.489, 118.007) -> (305.471, 118.163) projected
  line L1092 (305.496, 117.85) -> (305.489, 118.007) projected
  line L1093 (305.496, 2.1869) -> (305.496, 117.85) projected
  line L1094 (305.489, 2.0299) -> (305.496, 2.1869) projected
  line L1095 (305.471, 1.8741) -> (305.489, 2.0299) projected
  line L1096 (305.441, 1.7198) -> (305.471, 1.8741) projected
  line L1097 (305.398, 1.5696) -> (305.441, 1.7198) projected
  line L1098 (305.343, 1.4221) -> (305.398, 1.5696) projected
  line L1099 (305.278, 1.2788) -> (305.343, 1.4221) projected
  line L1100 (305.201, 1.1424) -> (305.278, 1.2788) projected
  line L1101 (305.114, 1.0115) -> (305.201, 1.1424) projected
  line L1102 (305.016, 0.8875) -> (305.114, 1.0115) projected
  line L1103 (304.91, 0.7731) -> (305.016, 0.8875) projected
  line L1104 (304.794, 0.6656) -> (304.91, 0.7731) projected
  line L1105 (304.672, 0.5691) -> (304.794, 0.6656) projected
  line L1106 (304.541, 0.4823) -> (304.672, 0.5691) projected
  line L1107 (304.403, 0.4051) -> (304.541, 0.4823) projected
  line L1108 (304.261, 0.339) -> (304.403, 0.4051) projected
  line L1109 (304.115, 0.2853) -> (304.261, 0.339) projected
  line L1110 (303.962, 0.2425) -> (304.115, 0.2853) projected
  line L1111 (303.808, 0.2122) -> (303.962, 0.2425) projected
  line L1112 (303.652, 0.1929) -> (303.808, 0.2122) projected
  line L1113 (303.496, 0.1874) -> (303.652, 0.1929) projected
  line L1114 (2.096, 0.1874) -> (303.496, 0.1874) projected
  line L1115 (1.9389, 0.1929) -> (2.096, 0.1874) projected
  line L1116 (1.7818, 0.2122) -> (1.9389, 0.1929) projected
  line L1117 (1.6288, 0.2425) -> (1.7818, 0.2122) projected
  line L1118 (1.4759, 0.2853) -> (1.6288, 0.2425) projected
  line L1119 (1.3298, 0.339) -> (1.4759, 0.2853) projected
  line L1120 (1.1879, 0.4051) -> (1.3298, 0.339) projected
  line L1121 (1.0501, 0.4823) -> (1.1879, 0.4051) projected
  line L1122 (0.9192, 0.5691) -> (1.0501, 0.4823) projected
  line L1123 (0.7965, 0.6656) -> (0.9192, 0.5691) projected
  line L1124 (0.6808, 0.7731) -> (0.7965, 0.6656) projected
  line L1125 (0.5746, 0.8875) -> (0.6808, 0.7731) projected
  line L1126 (0.4768, 1.0115) -> (0.5746, 0.8875) projected
  line L1127 (0.39, 1.1424) -> (0.4768, 1.0115) projected
  line L1128 (0.3128, 1.2788) -> (0.39, 1.1424) projected
  line L1129 (0.248, 1.4221) -> (0.3128, 1.2788) projected
  line L1130 (0.1929, 1.5696) -> (0.248, 1.4221) projected
  line L1131 (0.1502, 1.7198) -> (0.1929, 1.5696) projected
  line L1132 (0.1199, 1.8741) -> (0.1502, 1.7198) projected
  line L1133 (0.102, 2.0299) -> (0.1199, 1.8741) projected
  line L1134 (0.0951, 2.1869) -> (0.102, 2.0299) projected
  line L1135 (0.0951, 117.85) -> (0.0951, 2.1869) projected
  line L1136 (0.102, 118.007) -> (0.0951, 117.85) projected
  line L1137 (0.1199, 118.163) -> (0.102, 118.007) projected
  line L1138 (0.1502, 118.317) -> (0.1199, 118.163) projected
  line L1139 (0.1929, 118.468) -> (0.1502, 118.317) projected
  line L1140 (0.248, 118.616) -> (0.1929, 118.468) projected
  line L1141 (0.3128, 118.758) -> (0.248, 118.616) projected
  line L1142 (0.39, 118.894) -> (0.3128, 118.758) projected
  line L1143 (0.4768, 119.025) -> (0.39, 118.894) projected
  line L1144 (0.5746, 119.149) -> (0.4768, 119.025) projected
  line L1145 (0.6808, 119.265) -> (0.5746, 119.149) projected
  line L1146 (0.7965, 119.371) -> (0.6808, 119.265) projected
  line L1147 (0.9192, 119.469) -> (0.7965, 119.371) projected
  line L1148 (1.0501, 119.556) -> (0.9192, 119.469) projected
  line L1149 (1.1879, 119.633) -> (1.0501, 119.556) projected
  line L1150 (1.3298, 119.698) -> (1.1879, 119.633) projected
  line L1151 (1.4759, 119.753) -> (1.3298, 119.698) projected
  line L1152 (1.6288, 119.796) -> (1.4759, 119.753) projected
  line L1153 (1.7818, 119.826) -> (1.6288, 119.796) projected
  line L1154 (1.9389, 119.844) -> (1.7818, 119.826) projected
  line L1155 (2.096, 119.849) -> (1.9389, 119.844) projected
  line L1156 (288.771, 79.3129) -> (288.771, 93.1125) projected
  line L1157 (302.57, 79.3129) -> (288.771, 79.3129) projected
  line L1158 (302.57, 93.1125) -> (302.57, 79.3129) projected
  line L1159 (288.771, 93.1125) -> (302.57, 93.1125) projected
  line L1160 (243.527, 35.9625) -> (257.327, 35.9625) projected
  line L1161 (243.527, 22.163) -> (243.527, 35.9625) projected
  line L1162 (257.327, 22.163) -> (243.527, 22.163) projected
  line L1163 (257.327, 35.9625) -> (257.327, 22.163) projected
  line L1164 (302.57, 60.2629) -> (288.771, 60.2629) projected
  line L1165 (302.57, 74.0625) -> (302.57, 60.2629) projected
  line L1166 (288.771, 74.0625) -> (302.57, 74.0625) projected
  line L1167 (288.771, 60.2629) -> (288.771, 74.0625) projected
  line L1168 (250.671, 16.9127) -> (264.47, 16.9127) projected
  line L1169 (250.671, 3.113) -> (250.671, 16.9127) projected
  line L1170 (264.47, 3.113) -> (250.671, 3.113) projected
  line L1171 (264.47, 16.9127) -> (264.47, 3.113) projected
  line L1172 (219.713, 16.9127) -> (233.514, 16.9127) projected
  line L1173 (219.713, 3.113) -> (219.713, 16.9127) projected
  line L1174 (233.514, 3.113) -> (219.713, 3.113) projected
  line L1175 (233.514, 16.9127) -> (233.514, 3.113) projected
  line L1176 (302.57, 41.2129) -> (288.771, 41.2129) projected
  line L1177 (302.57, 55.0125) -> (302.57, 41.2129) projected
  line L1178 (288.771, 55.0125) -> (302.57, 55.0125) projected
  line L1179 (288.771, 41.2129) -> (288.771, 55.0125) projected
  line L1180 (288.771, 16.9127) -> (302.57, 16.9127) projected
  line L1181 (288.771, 3.113) -> (288.771, 16.9127) projected
  line L1182 (302.57, 3.113) -> (288.771, 3.113) projected
  line L1183 (302.57, 16.9127) -> (302.57, 3.113) projected
  line L1184 (269.721, 16.9127) -> (283.52, 16.9127) projected
  line L1185 (269.721, 3.113) -> (269.721, 16.9127) projected
  line L1186 (283.52, 3.113) -> (269.721, 3.113) projected
  line L1187 (283.52, 16.9127) -> (283.52, 3.113) projected
  line L1188 (283.52, 22.163) -> (269.721, 22.163) projected
  line L1189 (283.52, 35.9625) -> (283.52, 22.163) projected
  line L1190 (269.721, 35.9625) -> (283.52, 35.9625) projected
  line L1191 (269.721, 22.163) -> (269.721, 35.9625) projected
  line L1192 (288.771, 35.9625) -> (302.57, 35.9625) projected
  line L1193 (288.771, 22.163) -> (288.771, 35.9625) projected
  line L1194 (302.57, 22.163) -> (288.771, 22.163) projected
  line L1195 (302.57, 35.9625) -> (302.57, 22.163) projected
  line L1196 (59.6829, 35.9625) -> (59.6829, 22.163) projected
  line L1197 (45.8833, 35.9625) -> (59.6829, 35.9625) projected
  line L1198 (45.8833, 22.163) -> (45.8833, 35.9625) projected
  line L1199 (59.6829, 22.163) -> (45.8833, 22.163) projected
  line L1200 (5.4019, 16.9127) -> (19.2016, 16.9127) projected
  line L1201 (5.4019, 3.113) -> (5.4019, 16.9127) projected
  line L1202 (19.2016, 3.113) -> (5.4019, 3.113) projected
  line L1203 (19.2016, 16.9127) -> (19.2016, 3.113) projected
  line L1204 (29.213, 16.9127) -> (43.0142, 16.9127) projected
  line L1205 (29.213, 3.113) -> (29.213, 16.9127) projected
  line L1206 (43.0142, 3.113) -> (29.213, 3.113) projected
  line L1207 (43.0142, 16.9127) -> (43.0142, 3.113) projected
  line L1208 (145.408, 55.0125) -> (145.408, 41.2129) projected
  line L1209 (131.608, 55.0125) -> (145.408, 55.0125) projected
  line L1210 (131.608, 41.2129) -> (131.608, 55.0125) projected
  line L1211 (145.408, 41.2129) -> (131.608, 41.2129) projected
  line L1212 (164.458, 41.2129) -> (150.658, 41.2129) projected
  line L1213 (164.458, 55.0125) -> (164.458, 41.2129) projected
  line L1214 (150.658, 55.0125) -> (164.458, 55.0125) projected
  line L1215 (150.658, 41.2129) -> (150.658, 55.0125) projected
  line L1216 (273.995, 103.125) -> (260.196, 103.125) projected
  line L1217 (273.995, 116.926) -> (273.995, 103.125) projected
  line L1218 (260.196, 116.926) -> (273.995, 116.926) projected
  line L1219 (260.196, 103.125) -> (260.196, 116.926) projected
  line L1220 (241.146, 74.0625) -> (254.945, 74.0625) projected
  line L1221 (241.146, 60.2629) -> (241.146, 74.0625) projected
  line L1222 (254.945, 60.2629) -> (241.146, 60.2629) projected
  line L1223 (254.945, 74.0625) -> (254.945, 60.2629) projected
  line L1224 (254.945, 103.125) -> (241.146, 103.125) projected
  line L1225 (254.945, 116.926) -> (254.945, 103.125) projected
  line L1226 (241.146, 116.926) -> (254.945, 116.926) projected
  line L1227 (241.146, 103.125) -> (241.146, 116.926) projected
  line L1228 (235.895, 103.125) -> (222.096, 103.125) projected
  line L1229 (235.895, 116.926) -> (235.895, 103.125) projected
  line L1230 (222.096, 116.926) -> (235.895, 116.926) projected
  line L1231 (222.096, 103.125) -> (222.096, 116.926) projected
  line L1232 (245.42, 79.3129) -> (231.621, 79.3129) projected
  line L1233 (245.42, 93.1125) -> (245.42, 79.3129) projected
  line L1234 (231.621, 93.1125) -> (245.42, 93.1125) projected
  line L1235 (231.621, 79.3129) -> (231.621, 93.1125) projected
  line L1236 (226.37, 79.3129) -> (212.571, 79.3129) projected
  line L1237 (226.37, 93.1125) -> (226.37, 79.3129) projected
  line L1238 (212.571, 93.1125) -> (226.37, 93.1125) projected
  line L1239 (212.571, 79.3129) -> (212.571, 93.1125) projected
  line L1240 (217.333, 35.9625) -> (231.133, 35.9625) projected
  line L1241 (217.333, 22.163) -> (217.333, 35.9625) projected
  line L1242 (231.133, 22.163) -> (217.333, 22.163) projected
  line L1243 (231.133, 35.9625) -> (231.133, 22.163) projected
  line L1244 (198.283, 35.9625) -> (212.083, 35.9625) projected
  line L1245 (198.283, 22.163) -> (198.283, 35.9625) projected
  line L1246 (212.083, 22.163) -> (198.283, 22.163) projected
  line L1247 (212.083, 35.9625) -> (212.083, 22.163) projected
  line L1248 (235.895, 60.2629) -> (222.096, 60.2629) projected
  line L1249 (235.895, 74.0625) -> (235.895, 60.2629) projected
  line L1250 (222.096, 74.0625) -> (235.895, 74.0625) projected
  line L1251 (222.096, 60.2629) -> (222.096, 74.0625) projected
  line L1252 (193.033, 103.125) -> (179.233, 103.125) projected
  line L1253 (193.033, 116.926) -> (193.033, 103.125) projected
  line L1254 (179.233, 116.926) -> (193.033, 116.926) projected
  line L1255 (179.233, 103.125) -> (179.233, 116.926) projected
  line L1256 (216.845, 103.125) -> (203.046, 103.125) projected
  line L1257 (216.845, 116.926) -> (216.845, 103.125) projected
  line L1258 (203.046, 116.926) -> (216.845, 116.926) projected
  line L1259 (203.046, 103.125) -> (203.046, 116.926) projected
  line L1260 (216.845, 74.0625) -> (216.845, 60.2629) projected
  line L1261 (203.046, 74.0625) -> (216.845, 74.0625) projected
  line L1262 (203.046, 60.2629) -> (203.046, 74.0625) projected
  line L1263 (216.845, 60.2629) -> (203.046, 60.2629) projected
  line L1264 (207.32, 79.3129) -> (193.521, 79.3129) projected
  line L1265 (207.32, 93.1125) -> (207.32, 79.3129) projected
  line L1266 (193.521, 93.1125) -> (207.32, 93.1125) projected
  line L1267 (193.521, 79.3129) -> (193.521, 93.1125) projected
  line L1268 (188.27, 79.3129) -> (174.471, 79.3129) projected
  line L1269 (188.27, 93.1125) -> (188.27, 79.3129) projected
  line L1270 (174.471, 93.1125) -> (188.27, 93.1125) projected
  line L1271 (174.471, 79.3129) -> (174.471, 93.1125) projected
  line L1272 (183.508, 55.0125) -> (183.508, 41.2129) projected
  line L1273 (169.708, 55.0125) -> (183.508, 55.0125) projected
  line L1274 (169.708, 41.2129) -> (169.708, 55.0125) projected
  line L1275 (183.508, 41.2129) -> (169.708, 41.2129) projected
  line L1276 (197.795, 60.2629) -> (183.996, 60.2629) projected
  line L1277 (197.795, 74.0625) -> (197.795, 60.2629) projected
  line L1278 (183.996, 74.0625) -> (197.795, 74.0625) projected
  line L1279 (183.996, 60.2629) -> (183.996, 74.0625) projected
  line L1280 (178.745, 74.0625) -> (178.745, 60.2629) projected
  line L1281 (164.946, 74.0625) -> (178.745, 74.0625) projected
  line L1282 (164.946, 60.2629) -> (164.946, 74.0625) projected
  line L1283 (178.745, 60.2629) -> (164.946, 60.2629) projected
  line L1284 (154.933, 103.125) -> (141.133, 103.125) projected
  line L1285 (154.933, 116.926) -> (154.933, 103.125) projected
  line L1286 (141.133, 116.926) -> (154.933, 116.926) projected
  line L1287 (141.133, 103.125) -> (141.133, 116.926) projected
  line L1288 (173.983, 103.125) -> (160.183, 103.125) projected
  line L1289 (173.983, 116.926) -> (173.983, 103.125) projected
  line L1290 (160.183, 116.926) -> (173.983, 116.926) projected
  line L1291 (160.183, 103.125) -> (160.183, 116.926) projected
  line L1292 (169.22, 79.3129) -> (155.421, 79.3129) projected
  line L1293 (169.22, 93.1125) -> (169.22, 79.3129) projected
  line L1294 (155.421, 93.1125) -> (169.22, 93.1125) projected
  line L1295 (155.421, 79.3129) -> (155.421, 93.1125) projected
  line L1296 (150.17, 79.3129) -> (136.371, 79.3129) projected
  line L1297 (150.17, 93.1125) -> (150.17, 79.3129) projected
  line L1298 (136.371, 93.1125) -> (150.17, 93.1125) projected
  line L1299 (136.371, 79.3129) -> (136.371, 93.1125) projected
  line L1300 (260.196, 79.3129) -> (260.196, 84.0133) projected
  line L1301 (273.995, 79.3129) -> (260.196, 79.3129) projected
  line L1302 (273.995, 84.0133) -> (273.995, 79.3129) projected
  line L1303 (275.721, 84.0133) -> (273.995, 84.0133) projected
  line L1304 (275.721, 79.5433) -> (275.721, 84.0133) projected
  line L1305 (277.446, 79.5433) -> (275.721, 79.5433) projected
  line L1306 (277.446, 78.3428) -> (277.446, 79.5433) projected
  line L1307 (280.545, 78.3428) -> (277.446, 78.3428) projected
  line L1308 (280.545, 79.5433) -> (280.545, 78.3428) projected
  line L1309 (282.271, 79.5433) -> (280.545, 79.5433) projected
  line L1310 (282.271, 85.8132) -> (282.271, 79.5433) projected
  line L1311 (283.096, 85.8132) -> (282.271, 85.8132) projected
  line L1312 (283.096, 88.4135) -> (283.096, 85.8132) projected
  line L1313 (282.271, 88.4135) -> (283.096, 88.4135) projected
  line L1314 (282.271, 91.6421) -> (282.271, 88.4135) projected
  line L1315 (275.721, 91.6421) -> (282.271, 91.6421) projected
  line L1316 (275.721, 88.4135) -> (275.721, 91.6421) projected
  line L1317 (273.995, 88.4135) -> (275.721, 88.4135) projected
  line L1318 (273.995, 93.1125) -> (273.995, 88.4135) projected
  line L1319 (260.196, 93.1125) -> (273.995, 93.1125) projected
  line L1320 (260.196, 88.4135) -> (260.196, 93.1125) projected
  line L1321 (258.47, 88.4135) -> (260.196, 88.4135) projected
  line L1322 (258.47, 91.6421) -> (258.47, 88.4135) projected
  line L1323 (251.92, 91.6421) -> (258.47, 91.6421) projected
  line L1324 (251.92, 88.4135) -> (251.92, 91.6421) projected
  line L1325 (251.095, 88.4135) -> (251.92, 88.4135) projected
  line L1326 (251.095, 85.8132) -> (251.095, 88.4135) projected
  line L1327 (251.92, 85.8132) -> (251.095, 85.8132) projected
  line L1328 (251.92, 79.5433) -> (251.92, 85.8132) projected
  line L1329 (253.646, 79.5433) -> (251.92, 79.5433) projected
  line L1330 (253.646, 78.3428) -> (253.646, 79.5433) projected
  line L1331 (256.745, 78.3428) -> (253.646, 78.3428) projected
  line L1332 (256.745, 79.5433) -> (256.745, 78.3428) projected
  line L1333 (258.47, 79.5433) -> (256.745, 79.5433) projected
  line L1334 (258.47, 84.0133) -> (258.47, 79.5433) projected
  line L1335 (260.196, 84.0133) -> (258.47, 84.0133) projected
  line L1336 (278.758, 60.2629) -> (264.958, 60.2629) projected
  line L1337 (278.758, 74.0625) -> (278.758, 60.2629) projected
  line L1338 (264.958, 74.0625) -> (278.758, 74.0625) projected
  line L1339 (264.958, 60.2629) -> (264.958, 74.0625) projected
  line L1340 (257.813, 55.0125) -> (271.614, 55.0125) projected
  line L1341 (257.813, 50.3135) -> (257.813, 55.0125) projected
  line L1342 (256.089, 50.3135) -> (257.813, 50.3135) projected
  line L1343 (256.089, 53.5421) -> (256.089, 50.3135) projected
  line L1344 (249.538, 53.5421) -> (256.089, 53.5421) projected
  line L1345 (249.538, 50.3135) -> (249.538, 53.5421) projected
  line L1346 (248.714, 50.3135) -> (249.538, 50.3135) projected
  line L1347 (248.714, 47.7132) -> (248.714, 50.3135) projected
  line L1348 (249.538, 47.7132) -> (248.714, 47.7132) projected
  line L1349 (249.538, 41.4433) -> (249.538, 47.7132) projected
  line L1350 (251.263, 41.4433) -> (249.538, 41.4433) projected
  line L1351 (251.263, 40.2428) -> (251.263, 41.4433) projected
  line L1352 (254.362, 40.2428) -> (251.263, 40.2428) projected
  line L1353 (254.362, 41.4433) -> (254.362, 40.2428) projected
  line L1354 (256.089, 41.4433) -> (254.362, 41.4433) projected
  line L1355 (256.089, 45.9133) -> (256.089, 41.4433) projected
  line L1356 (257.813, 45.9133) -> (256.089, 45.9133) projected
  line L1357 (257.813, 41.2129) -> (257.813, 45.9133) projected
  line L1358 (271.614, 41.2129) -> (257.813, 41.2129) projected
  line L1359 (271.614, 45.9133) -> (271.614, 41.2129) projected
  line L1360 (273.338, 45.9133) -> (271.614, 45.9133) projected
  line L1361 (273.338, 41.4433) -> (273.338, 45.9133) projected
  line L1362 (275.063, 41.4433) -> (273.338, 41.4433) projected
  line L1363 (275.063, 40.2428) -> (275.063, 41.4433) projected
  line L1364 (278.164, 40.2428) -> (275.063, 40.2428) projected
  line L1365 (278.164, 41.4433) -> (278.164, 40.2428) projected
  line L1366 (279.888, 41.4433) -> (278.164, 41.4433) projected
  line L1367 (279.888, 47.7132) -> (279.888, 41.4433) projected